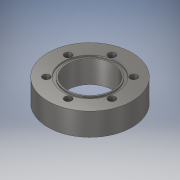
# Autodesk Inventor part: adapter
Saved by Autodesk Inventor 2018 (Build 220112000, 112)
## iProperties
Created: 2019-03-04
Part Number: adapter
Material: Stainless Steel
Document SubType Name: Modeling
Designer: Admin
Density: 8 g/cm^3
Appearance: Semi-Polished
Author: Admin
Autodesk Inventor part; units mm, degrees
ref_plane "YZ Plane" through (0, 0, 0) normal (1, 0, 0) x (0, 1, 0)
ref_plane "XZ Plane" through (0, 0, 0) normal (0, 1, 0) x (-1, 0, 0)
ref_plane "XY Plane" through (0, 0, 0) normal (0, 0, 1) x (1, 0, 0)
sketch "Sketch1" plane through (0, 0, 0) normal (0, 1, 0) x (-1, 0, 0)
  circle A0 centre (0, 0) radius 23.495
  dimension "d0" = 46.99
  constraints: 1 centre point, 1 coincident
  measures "d0" diameter of A0
extrude "Extrusion1" add sketch "Sketch1" along normal blind 12.7
sketch "Sketch2" plane through (0, 0, 0) normal (0, -1, 0) x (1, 0, 0)
  circle A0 centre (0, 0) radius 22.733
  circle A1 centre (0, 0) radius 23.495 projected
  circle A2 centre (0, 0) radius 21.209
  dimension "d3" = 0.762
  dimension "d4" = 1.524
  constraints: 2 centre point, 2 coincident
  measures "d3" radial gap between concentric circles of A1 A0
  measures "d4" radial gap between concentric circles of A0 A2
extrude "Extrusion2" cut sketch "Sketch2" against normal blind 0.762 contours A0
sketch "Sketch3" plane through (0, 12.7, 0) normal (0, 1, 0) x (1, 0, 0)
  circle A0 centre (0, 0) radius 12.7
  dimension "d7" = 25.4
  constraints: 1 centre point, 1 coincident
  measures "d7" diameter of A0
extrude "Extrusion3" cut sketch "Sketch3" against normal up to surface (12.7 mm away)
sketch "Sketch4" plane through (0, 12.7, 0) normal (0, 1, 0) x (1, 0, 0)
  circle A0 centre (0, 0) radius 13.462
  circle A1 centre (0, 0) radius 12.7 projected
  circle A2 centre (0, 0) radius 14.986
  dimension "d10" = 0.762
  dimension "d11" = 1.524
  constraints: 2 centre point, 2 coincident
  measures "d10" radial gap between concentric circles of A0 A1
  measures "d11" radial gap between concentric circles of A2 A0
extrude "Extrusion4" cut sketch "Sketch4" against normal blind 0.762 contours A2
sketch "Sketch5" plane through (0, 0, 0) normal (0, -1, 0) x (1, 0, 0)
  line L0 (0, 0) -> (12.2131, -12.2131) construction
  line L1 (0, 0) -> (17.272, 0) construction
  dimension "d14" = 17.272
  dimension "d15" = 45
  constraints: 4 end point, 1 coincident, 1 equal length, 1 horizontal
  measures "d14" distance of L0.start L0.end
  measures "d15" angle of L0 L1
hole "Hole1" at (12.2131, 0, -12.2131) direction (0, 1, 0) diameter 3.9624 depth 13.6144 tip angle 118 thread size "10-32 UNF" class "2B" standard "ANSI Unified Screw Threads"
chamfer "Chamfer1" distance 0.381 angle 45 1 edges at (12.2131, 0, -10.2319)
pattern_circular "Circular Pattern1" count 6 over 360 about axis through (0, 0, 0) along (0, 1, 0) of "Hole1", "Chamfer1"
body "Solid1"
